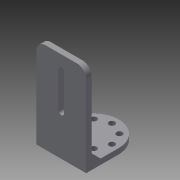
# Autodesk Inventor part: c920_plate
Saved by Autodesk Inventor 2013 (Build 170138000, 138)
## iProperties
Created: 2013-03-18
Part Number: c920_plate
Material: Generic
Document SubType Name: Modeling
Designer: Mahisorn
Density: 1 g/cm^3
Author: Mahisorn
Autodesk Inventor part; units mm, degrees
ref_plane "YZ Plane" through (0, 0, 0) normal (1, 0, 0) x (0, 1, 0)
ref_plane "XZ Plane" through (0, 0, 0) normal (0, 1, 0) x (-1, 0, 0)
ref_plane "XY Plane" through (0, 0, 0) normal (0, 0, 1) x (1, 0, 0)
sketch "Sketch1" plane through (0, 0, 0) normal (0, 0, 1) x (1, 0, 0)
  circle A0 centre (0, 0) radius 27.5
  line L0 (-27.5, 0) -> (27.5, 0)
  line L1 (27.5, 0) -> (27.5, -36)
  line L2 (27.5, -36) -> (-27.5, -36)
  line L3 (-27.5, -36) -> (-27.5, 0)
  line L4 (27.5, -30) -> (-27.5, -30)
  point P0 (20, 0)
  point P1 (20, 0)
  point P2 (20, 0)
  dimension "d0" = 55
  dimension "d1" = 36
  dimension "d2" = 6
  dimension "d7" = 20
  constraints: 10 end point, 5 coincident, 3 point on line, 2 parallel, 2 perpendicular, 1 horizontal, 1 horizontal alignment, 2 other
  measures "d1" distance of L0.end L1.end
  measures "d2" distance between parallel lines of L2 L4
  measures "d7" distance of point (20, 0) point (0, 0)
extrude "Extrusion1" add sketch "Sketch1" along normal blind 6 contours L0 A0 | L1 L4 L3 A0 | A0 L0
extrude "Extrusion2" add sketch "Sketch1" along normal blind 100 contours L1 L2 L3 L4
sketch "Sketch2" plane through (0, 0, 6) normal (0, 0, 1) x (1, 0, 0)
  arc A0 (27.5, 0) -> (-27.5, 0) centre (0, 0) ccw projected
  line L0 (-27.5, -30) -> (-21.5, -30)
  line L1 (-21.5, -30) -> (-21.5, -20)
  line L2 (-21.5, -20) -> (-27.5, -20)
  line L3 (-27.5, -20) -> (-27.5, -30)
  point P0 (20, 0)
  point P1 (14.1421, 14.1421)
  point P2 (0, 20)
  point P3 (-14.1421, 14.1421)
  point P4 (-20, 0)
  point P5 (-14.1421, -14.1421)
  point P6 (0, -20)
  point P7 (14.1421, -14.1421)
  dimension "d8" = 20
  dimension "d11" = 360
  dimension "d20" = 6
  dimension "d21" = 10
  constraints: 8 end point, 2 parallel, 1 horizontal, 1 perpendicular, 9 other
  measures "d8" distance of point (20, 0) A0.centre
  measures "d20" distance of L2.end L1.end
  measures "d21" distance of L1.end L0.end
hole "Hole1" at (20, 0, 6) at (0, 20, 6) at (-14.1421, 14.1421, 6) at (-20, 0, 6) at (-14.1421, -14.1421, 6) at (0, -20, 6) at (14.1421, -14.1421, 6) at (14.1421, 14.1421, 6) direction (0, 0, -1) diameter 6.6 end through all clearance for "Flat Head Machine Screw" size "M6" standard "Ansi Metric M Profile"
extrude "Extrusion3" add sketch "Sketch2" along normal blind 10
mirror "Mirror3" about plane through (0, 0, 0) normal (1, 0, 0) of "Extrusion3"
chamfer "Chamfer1" distance 10 angle 45 2 edges at (-24.5, -20, 16) (24.5, -20, 16)
sketch "Sketch3" plane through (-27.5, -30, 100) normal (0, 1, 0) x (1, 0, 0)
  line L0 (55, 0) -> (0, 0) projected
  line L1 (55, 84) -> (55, 0) projected
  arc A0 (30.65, 55) -> (24.35, 55) centre (27.5, 55) ccw
  arc A1 (24.35, 15) -> (30.65, 15) centre (27.5, 15) ccw
  line L2 (30.65, 55) -> (30.65, 15)
  line L3 (24.35, 55) -> (24.35, 15)
  point P0 (27.5, 100)
  dimension "d27" = 15
  dimension "d28" = 40
  dimension "d29" = 3.15
  dimension "d30" = 3.15
  constraints: 4 end point, 4 point on circle, 4 tangent, 2 centre point, 2 coincident, 1 parallel
  measures "d27" distance from line of L0 point (27.5, 15)
  measures "d28" distance of point (27.5, 15) point (27.5, 55)
  measures "d29" radius of A0
  measures "d30" radius of A1
extrude "Extrusion4" cut sketch "Sketch3" against normal through all
fillet "Fillet1" radius 10 2 edges at (27.5, -33, 100) (-27.5, -33, 100)
body "Solid1"
